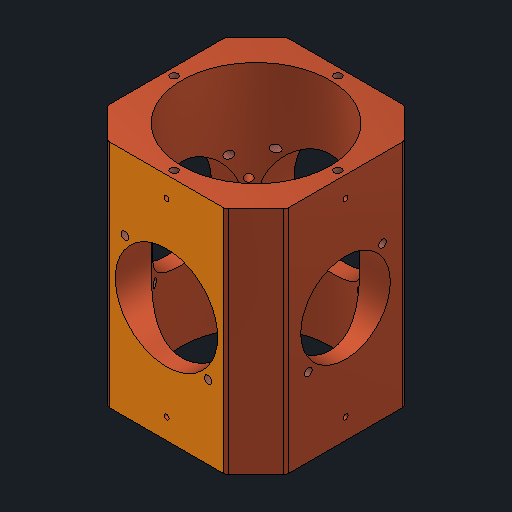
# Autodesk Inventor part: plasma_box
Saved by Autodesk Inventor 2025 (Build 290162000, 162)
## iProperties
Created: 2023-12-08
Part Number: plasma_box
Material: 銅
Document SubType Name: Modeling
Designer: Jinya H
Density: 8.94 g/cm^3
Appearance: 銅 - サテン
Author: Jinya H
Title: Plasma Box
Autodesk Inventor part; units mm, degrees
note: some values were not read from the file. Chosen so that the rebuilt part matches the saved one: direction of "Vacuum-vent".
ref_plane "YZ Plane" through (0, 0, 0) normal (1, 0, 0) x (0, 1, 0)
ref_plane "XZ Plane" through (0, 0, 0) normal (0, 1, 0) x (-1, 0, 0)
ref_plane "XY Plane" through (0, 0, 0) normal (0, 0, 1) x (1, 0, 0)
sketch "スケッチ1" plane through (0, 0, 0) normal (0, 1, 0) x (-1, 0, 0)
  line L0 (35, -35) -> (-35, -35)
  line L1 (-35, -35) -> (-35, 35)
  line L2 (-35, 35) -> (35, 35)
  line L3 (35, 35) -> (35, -35)
  line L4 (35, -35) -> (-35, 35) construction
  line L5 (-35, -35) -> (35, 35) construction
  point P0 (0, 0)
  dimension "d0" = 70
  dimension "d1" = 70
  constraints: 12 end point, 2 midpoint, 2 parallel, 1 horizontal, 1 perpendicular
  measures "d0" distance of L1.end L2.end
  measures "d1" distance of L0.end L1.end
extrude "Box" add sketch "スケッチ1" along normal mid plane 90
sketch "スケッチ2" plane through (-35, 45, 35) normal (0, 0, 1) x (1, 0, 0)
  circle A0 centre (35, -45) radius 20
  dimension "d4" = 40
  constraints: 1 centre point, 1 coincident
  measures "d4" diameter of A0
extrude "Probe-hole-40mm" cut sketch "スケッチ2" against normal through all
sketch "スケッチ3" plane through (35, -45, -35) normal (1, 0, 0) x (0, 0, -1)
  circle A0 centre (-35, 45) radius 17.5
  dimension "d7" = 35
  constraints: 1 centre point, 1 coincident
  measures "d7" diameter of A0
extrude "Diagnostic-hole-35mm" cut sketch "スケッチ3" against normal through all
sketch "スケッチ4" plane through (0, 45, 0) normal (0, 1, 0) x (1, 0, 0)
  line L0 (0, 0) -> (-20, -20) projected
  circle A0 centre (0, 0) radius 29
  dimension "d10" = 58
  constraints: 1 centre point, 1 coincident
  measures "d10" diameter of A0
extrude "Plasma-hole-58mm" cut sketch "スケッチ4" against normal through all
sketch "スケッチ5" plane through (0, 45, 0) normal (0, 1, 0) x (1, 0, 0)
  circle A0 centre (0, 0) radius 32 construction
  point P0 (32, 0)
  dimension "d164" = 64
  constraints: 2 horizontal alignment, 1 coincident, 2 other
hole "Connection-hole" at (32, 45, 0) direction (0, -1, 0) diameter 3 depth 10 tip angle 118
sketch "スケッチ7" plane through (35, -45, -35) normal (1, 0, 0) x (0, 0, -1)
  line L0 (0, 90) -> (-70, 90) projected
  line L1 (-36.5, 90) -> (-33.5, 90) projected
  line L2 (-33.5, 80) -> (-36.5, 80) projected
  line L3 (-33.5, 80) -> (-33.5, 90) projected
  line L4 (-36.5, 80) -> (-36.5, 90) projected
  line L5 (-36.5, 90) -> (-33.5, 90) projected
  point P0 (-35, 45)
  point P1 (-35, 82)
  point P2 (-35, 80)
  dimension "d173" = 2
  constraints: 1 midpoint, 1 vertical alignment
  measures "d173" distance from line of L2 point (-35, 82)
hole "Vacuum-vent" at (35, 37, 0) direction (-1, 0, 0) diameter 2 end up to surface
thread "Connection-thread" size "M3x0.5" class "6H" standard "ANSI Metric M Profile" full length
pattern_circular "Circular Pattern8" count 4 over 360 about axis through (0, 45, 0) along (0, -1, 0) of "Connection-hole", "Vacuum-vent"
mirror "Mirror1" about plane through (0, 0, 0) normal (0, 1, 0) of "Connection-hole", "Vacuum-vent", "Circular Pattern8"
chamfer "面取り3" distance 12 angle 45 4 edges at (35, 0, -35) (-35, 0, -35) (35, 0, 35) (-35, 0, 35)
fillet "フィレット3" radius 2 8 edges at (-23, 0, 35) (-35, 0, 23) (-35, 0, -23) (-23, 0, -35) (23, 0, -35) (35, 0, -23) (35, 0, 23) (23, 0, 35)
sketch "スケッチ17" plane through (-23.5858, -45, -34.4142) normal (-0.7071068, 0, -0.7071068) x (-0.7071068, 0, 0.7071068)
  line L0 (7.6569, 45) -> (9.6569, 45) construction
  line L1 (15.3137, 90) -> (15.3137, 0) projected
  circle A0 centre (9.6569, 39) radius 1.5
  circle A1 centre (9.6569, 51) radius 1.5
  dimension "d110" = 2
  dimension "d113" = 3
  constraints: 2 centre point, 2 end point, 1 perpendicular, 1 symmetric about line, 1 other
  measures "d110" distance of L0.start L0.end
  measures "d113" diameter of A0
extrude "Hinge-threads" cut sketch "スケッチ17" against normal blind 20
sketch "スケッチ18" plane through (-35, -45, -22.1716) normal (-1, 0, 0) x (0, 0, 1)
  arc A0 (42.6716, 45) -> (7.6759, 59.4957) centre (22.1716, 45) ccw construction
  line L0 (22.1716, 45) -> (7.6759, 59.4957) construction
  line L1 (22.1716, 45) -> (42.6716, 45) construction
  circle A1 centre (7.6759, 59.4957) radius 1.5
  circle A2 centre (36.6673, 30.5043) radius 1.5
  dimension "d138" = 20.5
  dimension "d139" = 135
  dimension "d140" = 3
  dimension "d143" = 360
  constraints: 4 end point, 3 centre point, 2 coincident, 2 point on circle, 1 equal length, 1 horizontal, 5 other
  measures "d138" radius of A0
  measures "d139" angle of L1 L0
  measures "d140" diameter of A1
extrude "Window-mounting-threads-1" cut sketch "スケッチ18" against normal through all
sketch "スケッチ19" plane through (-22.1716, 45, 35) normal (0, 0, 1) x (1, 0, 0)
  arc A0 (45.1716, -45) -> (5.9081, -28.7365) centre (22.1716, -45) ccw
  line L0 (22.1716, -45) -> (5.9081, -28.7365) construction
  line L1 (22.1716, -45) -> (45.1716, -45) construction
  circle A1 centre (5.9081, -28.7365) radius 1.5
  circle A2 centre (38.435, -61.2635) radius 1.5
  dimension "d155" = 23
  dimension "d156" = 135
  dimension "d157" = 3
  dimension "d160" = 360
  constraints: 4 end point, 3 centre point, 2 coincident, 2 point on circle, 5 other
  measures "d155" radius of A0
  measures "d156" angle of L1 L0
  measures "d157" diameter of A1
extrude "Window-mounting-threads-2" cut sketch "スケッチ19" against normal through all
thread "Thread16" size "M3x0.5" class "6H" standard "ANSI Metric M Profile" full length
thread "Thread17" size "M3x0.5" class "6H" standard "ANSI Metric M Profile" full length
thread "Thread18" size "M3x0.5" class "6H" standard "ANSI Metric M Profile" full length
thread "Thread19" size "M3x0.5" class "6H" standard "ANSI Metric M Profile" full length
thread "Thread20" size "M3x0.5" class "6H" standard "ANSI Metric M Profile" full length
thread "Thread21" size "M3x0.5" class "6H" standard "ANSI Metric M Profile" full length
thread "Thread22" size "M3x0.5" class "6H" standard "ANSI Metric M Profile" full length
thread "Thread23" size "M3x0.5" class "6H" standard "ANSI Metric M Profile" full length
